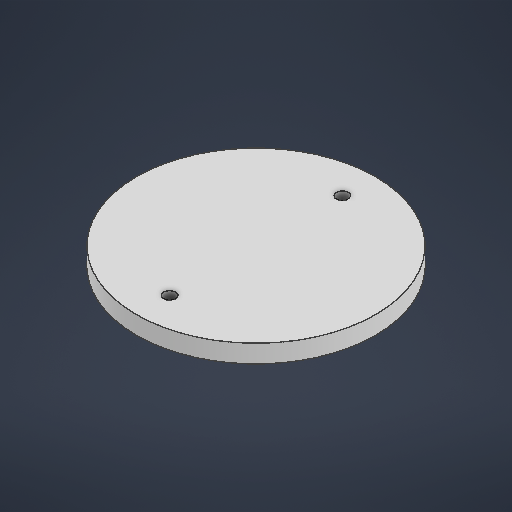
# Autodesk Inventor part: gearwheel_big
Saved by Autodesk Inventor 2026.1 (Build 301233000, 233)
## iProperties
Created: 2025-10-19
Part Number: gearwheel_big
Material: Generic
Document SubType Name: Modeling
Designer: emanuel
Density: 1 g/cm^3
Appearance: Default
Author: emanuel
Autodesk Inventor part; units mm, degrees
ref_plane "YZ Plane" through (0, 0, 0) normal (1, 0, 0) x (0, 1, 0)
ref_plane "XZ Plane" through (0, 0, 0) normal (0, 1, 0) x (-1, 0, 0)
ref_plane "XY Plane" through (0, 0, 0) normal (0, 0, 1) x (1, 0, 0)
sketch "Sketch1" plane through (0, 0, 0) normal (0, 1, 0) x (-1, 0, 0)
  circle A0 centre (0, 0) radius 16.05
  circle A1 centre (0, 0) radius 20
  line L0 (0, 16.05) -> (0, 14.5865)
  line L1 (0, 16.05) -> (0, 14.45)
  line L2 (0, 14.45) -> (0, -14.45)
  line L3 (0, -14.45) -> (0, -16.05)
  circle A2 centre (0, 14.45) radius 1
  circle A3 centre (0, -14.45) radius 1
  dimension "d0" = 32.1
  dimension "d1" = 40
  dimension "d2" = 1.6
  dimension "d3" = 28.9
  dimension "d4" = 2
  dimension "d5" = 2
  constraints: 8 end point, 4 centre point, 4 coincident, 2 point on circle, 2 point on line, 2 vertical
  measures "d0" diameter of A0
  measures "d1" diameter of A1
  measures "d2" distance of L0.start L1.end
  measures "d3" distance of L1.end L2.end
  measures "d4" diameter of A2
  measures "d5" diameter of A3
extrude "Extrusion1" add sketch "Sketch1" along normal blind 3 contours A0 L3 A3 L2 A2 L0 | L0 A2 L2 A3 L3 A0 | A1
body "Solid1"
